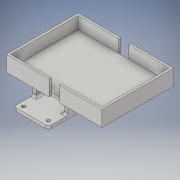
# Autodesk Inventor part: батарейки
Saved by Autodesk Inventor 2019.1 (Build 231200000, 200)
## iProperties
Created: 2021-01-12
Part Number: батарейки
Material: Типовые
Document SubType Name: Modeling
Designer: ученик
Density: 1 g/cm^3
Appearance: По умолчанию
Author: ученик
Autodesk Inventor part; units mm, degrees
ref_plane "YZ Plane" through (0, 0, 0) normal (1, 0, 0) x (0, 1, 0)
ref_plane "XZ Plane" through (0, 0, 0) normal (0, 1, 0) x (-1, 0, 0)
ref_plane "XY Plane" through (0, 0, 0) normal (0, 0, 1) x (1, 0, 0)
sketch "Эскиз1" plane through (0, 0, 0) normal (0, 1, 0) x (-1, 0, 0)
  circle A0 centre (16, 32.5) radius 1.75
  circle A1 centre (16, -17) radius 1.75
  circle A2 centre (-8, -17) radius 1.75
  circle A3 centre (-8, 32.5) radius 1.75
  line L0 (20.75, 37.25) -> (-12.75, 37.25)
  line L1 (-12.75, 37.25) -> (-12.75, -21.75)
  line L2 (-12.75, -21.75) -> (20.75, -21.75)
  line L3 (20.75, -21.75) -> (20.75, 37.25)
  point P0 (0, 0)
  dimension "d0" = 3.5
  dimension "d1" = 3.5
  dimension "d2" = 46
  dimension "d3" = 3.5
  dimension "d4" = 20.5
  dimension "d5" = 3.5
  dimension "d6" = 46
  dimension "d8" = 20.5
  dimension "d9" = 3
  dimension "d10" = 3
  dimension "d11" = 3
  dimension "d12" = 3
  dimension "d13" = 3
  dimension "d14" = 3
  dimension "d15" = 59
  dimension "d16" = 3
  dimension "d17" = 4.75
  constraints: 8 end point, 4 centre point, 2 parallel, 1 horizontal, 1 perpendicular
  measures "d0" diameter of A0
  measures "d1" diameter of A1
  measures "d3" diameter of A2
  measures "d5" diameter of A3
  measures "d9" distance edge to line of A0 L3
  measures "d10" distance edge to line of A0 L0
  measures "d11" distance edge to line of A3 L0
  measures "d12" distance edge to line of A3 L1
  measures "d13" distance edge to line of A1 L3
  measures "d14" distance edge to line of A1 L2
  measures "d15" distance of L0.end L1.end
  measures "d16" distance edge to line of A2 L2
  measures "d17" distance from line of A2.centre L1
extrude "Выдавливание1" add sketch "Эскиз1" along normal blind 3
sketch "Эскиз2" plane through (0, 3, 0) normal (0, 1, 0) x (1, 0, 0)
  line L0 (-20.75, 21.75) -> (-20.75, -37.25) projected
  line L1 (-20.75, 3.25) -> (-17.75, 3.25)
  line L2 (-17.75, 3.25) -> (-17.75, -18.75)
  line L3 (-17.75, -18.75) -> (-20.75, -18.75)
  line L4 (-20.75, -18.75) -> (-20.75, 3.25)
  line L5 (12.75, -37.25) -> (12.75, 21.75) projected
  line L6 (12.75, 3.25) -> (9.75, 3.25)
  line L7 (9.75, 3.25) -> (9.75, -18.75)
  line L8 (9.75, -18.75) -> (12.75, -18.75)
  line L9 (12.75, -18.75) -> (12.75, 3.25)
  line L10 (12.75, 21.75) -> (-20.75, 21.75) projected
  line L11 (-20.75, -37.25) -> (12.75, -37.25) projected
  point P0 (0, 0)
  dimension "d20" = 59
  dimension "d21" = 3
  dimension "d22" = 3
  dimension "d23" = 22
  dimension "d24" = 22
  dimension "d25" = 18.5
  dimension "d26" = 18.5
  dimension "d27" = 18.5
  constraints: 16 end point, 4 parallel, 2 horizontal, 2 perpendicular, 2 point on line
  measures "d20" distance of L0.start L0.end
  measures "d21" distance of L2.end L3.end
  measures "d22" distance of L7.end L8.end
  measures "d23" distance of L1.end L2.end
  measures "d24" distance of L6.end L7.end
  measures "d25" distance between parallel lines of L10 L1
  measures "d26" distance between parallel lines of L11 L3
  measures "d27" distance between parallel lines of L10 L6
extrude "Выдавливание2" add sketch "Эскиз2" along normal blind 30 contours L1 L2 L3 L0 | L5 L8 L7 L6
sketch "Эскиз3" plane through (0, 33, 0) normal (0, 1, 0) x (1, 0, 0)
  line L0 (-20.75, 21.75) -> (-20.75, 3.25) projected
  line L1 (-20.75, 24.75) -> (67.25, 24.75)
  line L2 (67.25, 24.75) -> (67.25, -40.25)
  line L3 (67.25, -40.25) -> (-20.75, -40.25)
  line L4 (-20.75, -40.25) -> (-20.75, 24.75)
  line L5 (12.75, 21.75) -> (-20.75, 21.75) projected
  line L6 (-20.75, -37.25) -> (12.75, -37.25) projected
  line L7 (69.25, 26.75) -> (-22.75, 26.75)
  line L8 (-22.75, 26.75) -> (-22.75, -42.25)
  line L9 (-22.75, -42.25) -> (69.25, -42.25)
  line L10 (69.25, -42.25) -> (69.25, 26.75)
  point P0 (0, 0)
  dimension "d30" = 88
  dimension "d31" = 65
  dimension "d34" = 59
  dimension "d35" = 88
  dimension "d38" = 3
  dimension "d39" = 2
  dimension "d40" = 2
  dimension "d41" = 2
  dimension "d42" = 2
  constraints: 16 end point, 4 parallel, 2 horizontal, 2 perpendicular, 1 point on line
  measures "d30" distance of L1.start L1.end
  measures "d31" distance of L1.end L2.end
  measures "d34" distance between parallel lines of L6 L5
  measures "d35" distance of L2.end L3.end
  measures "d38" distance between parallel lines of L6 L3
  measures "d39" distance between parallel lines of L10 L2
  measures "d40" distance between parallel lines of L9 L3
  measures "d41" distance between parallel lines of L7 L1
  measures "d42" distance between parallel lines of L4 L8
extrude "Выдавливание3" add sketch "Эскиз3" along normal blind 3 contours L4 L1 L2 L3 L0
sketch "Эскиз4" plane through (0, 36, 0) normal (0, 1, 0) x (1, 0, 0)
  line L0 (67.25, 24.75) -> (-20.75, 24.75) projected
  line L1 (67.25, 24.75) -> (-20.75, 24.75)
  line L2 (-20.75, 24.75) -> (-20.75, -40.25)
  line L3 (-20.75, -40.25) -> (67.25, -40.25)
  line L4 (67.25, -40.25) -> (67.25, 24.75)
  line L5 (69.25, 26.75) -> (-22.75, 26.75)
  line L6 (-22.75, 26.75) -> (-22.75, -42.25)
  line L7 (-22.75, -42.25) -> (69.25, -42.25)
  line L8 (69.25, -42.25) -> (69.25, 26.75)
  line L9 (33.25, 26.75) -> (23.25, 26.75)
  line L10 (23.25, 24.75) -> (33.25, 24.75)
  line L11 (67.25, -40.25) -> (-20.75, -40.25) projected
  line L12 (30, -42.25) -> (40, -42.25)
  line L13 (40, -40.25) -> (30, -40.25)
  line L14 (28.25, 24.75) -> (18.25, 24.75)
  line L15 (18.25, 24.75) -> (18.25, 26.75)
  line L16 (18.25, 26.75) -> (28.25, 26.75)
  line L17 (28.25, 26.75) -> (28.25, 24.75)
  line L18 (18.25, -40.25) -> (28.25, -40.25)
  line L19 (28.25, -40.25) -> (28.25, -42.25)
  line L20 (28.25, -42.25) -> (18.25, -42.25)
  line L21 (18.25, -42.25) -> (18.25, -40.25)
  point P0 (0, 0)
  dimension "d43" = 2
  dimension "d44" = 2
  dimension "d45" = 2
  dimension "d46" = 2
  dimension "d51" = 10
  dimension "d52" = 41
  dimension "d53" = 41
  dimension "d54" = 10
  dimension "d55" = 41
  constraints: 40 end point, 10 parallel, 6 horizontal, 6 point on line, 4 perpendicular, 2 midpoint
  measures "d43" distance between parallel lines of L8 L4
  measures "d44" distance between parallel lines of L7 L3
  measures "d45" distance between parallel lines of L5 L0
  measures "d46" distance between parallel lines of L2 L6
  measures "d51" distance between parallel lines of L15 L17
  measures "d52" distance between parallel lines of L8 L17
  measures "d53" distance between parallel lines of L15 L6
  measures "d54" distance between parallel lines of L21 L19
  measures "d55" distance between parallel lines of L6 L21
extrude "Выдавливание4" add sketch "Эскиз4" along normal blind 12 and the other way blind 3 contours L0 L17 L5 L8 L7 L19 L3 L4 | L0 L2 L3 L21 L7 L6 L5 L15
fillet "Сопряжение1" radius 2 3 edges at (9.75, 3, 7.75) (11.25, 3, 18.75) (11.25, 3, -3.25)
fillet "Сопряжение2" radius 2 3 edges at (-19.25, 3, -3.25) (-17.75, 3, 7.75) (-19.25, 3, 18.75)
fillet "Сопряжение3" radius 2 8 edges at (11.25, 33, 18.75) (12.75, 33, 7.75) (-17.75, 33, 7.75) (-19.25, 33, 18.75) (-20.75, 33, 7.75) (-19.25, 33, -3.25) (9.75, 33, 7.75) (11.25, 33, -3.25)
fillet "Сопряжение4" radius 3 4 edges at (-20.75, 1.5, 37.25) (12.75, 1.5, 37.25) (-20.75, 1.5, -21.75) (12.75, 1.5, -21.75)
